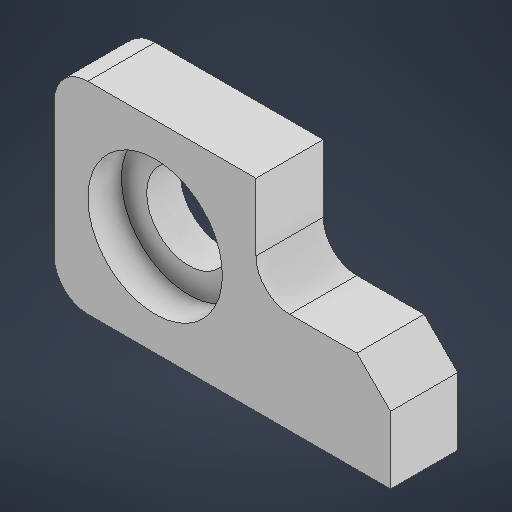
# Autodesk Inventor part: Part6
Saved by Autodesk Inventor 2026 (Build 300175050, 175E)
## iProperties
Created: 2026-03-19
Part Number: Part6
Material: Generic
Document SubType Name: Modeling
Designer: Administrator
Density: 1 g/cm^3
Appearance: Default
Author: Administrator
Autodesk Inventor part; units mm, degrees
ref_plane "YZ Plane" through (0, 0, 0) normal (1, 0, 0) x (0, 1, 0)
ref_plane "XZ Plane" through (0, 0, 0) normal (0, 1, 0) x (-1, 0, 0)
ref_plane "XY Plane" through (0, 0, 0) normal (0, 0, 1) x (1, 0, 0)
sketch "Sketch2" plane through (0, 0, 0) normal (0, 0, 1) x (1, 0, 0)
  line L0 (0, 0) -> (100, 0)
  line L1 (100, 0) -> (100, 30)
  line L2 (100, 30) -> (60, 30)
  line L3 (60, 30) -> (60, 60)
  line L4 (60, 60) -> (0, 60)
  line L5 (0, 60) -> (0, 0)
  dimension "d0" = 30
  dimension "d1" = 100
  dimension "d2" = 40
  dimension "d3" = 60
  constraints: 12 end point, 5 perpendicular, 1 horizontal
  measures "d0" distance of L0.end L1.end
  measures "d1" distance of L0.start L0.end
  measures "d2" distance of L1.end L2.end
  measures "d3" distance of L4.end L0.start
extrude "Extrusion1" add sketch "Sketch2" along normal mid plane 20
fillet "Fillet1" radius 10 1 edges at (60, 30, 0)
fillet "Fillet2" radius 10 1 edges at (0, 60, 0)
fillet "Fillet3" radius 10 1 edges at (0, 0, 0)
chamfer "Chamfer1" distance 10 angle 45 1 edges at (100, 30, 0)
sketch "Sketch3" plane through (0, 0, 10) normal (0, 0, 1) x (1, 0, 0)
  circle A0 centre (30, 30) radius 12.5
  line L0 (10, 0) -> (100, 0) projected
  line L1 (0, 50) -> (0, 10) projected
  point P0 (0, 0)
  dimension "d12" = 25
  dimension "d13" = 30
  dimension "d14" = 30
  constraints: 1 centre point
  measures "d12" diameter of A0
  measures "d13" distance from line of L0 A0.centre
  measures "d14" distance from line of L1 A0.centre
extrude "Extrusion2" cut sketch "Sketch3" against normal blind 20
sketch "Sketch4" plane through (0, 0, 10) normal (0, 0, 1) x (1, 0, 0)
  circle A0 centre (30, 30) radius 20
  line L0 (10, 0) -> (100, 0) projected
  line L1 (0, 50) -> (0, 10) projected
  point P0 (0, 0)
  dimension "d17" = 40
  dimension "d18" = 30
  dimension "d19" = 30
  constraints: 1 centre point
  measures "d17" diameter of A0
  measures "d18" distance from line of L0 A0.centre
  measures "d19" distance from line of L1 A0.centre
extrude "Extrusion3" cut sketch "Sketch4" against normal blind 10
body "Solid1"
